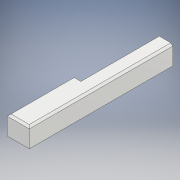
# Autodesk Inventor part: key_2
Saved by Autodesk Inventor 2017 (Build 210142000, 142)
## iProperties
Created: 2018-03-15
Part Number: key_2
Material: Generic
Document SubType Name: Modeling
Designer: Luiz Gustavo
Density: 1 g/cm^3
Appearance: White
Author: Luiz Gustavo
Autodesk Inventor part; units mm, degrees
ref_plane "YZ Plane" through (0, 0, 0) normal (1, 0, 0) x (0, 1, 0)
ref_plane "XZ Plane" through (0, 0, 0) normal (0, 1, 0) x (-1, 0, 0)
ref_plane "XY Plane" through (0, 0, 0) normal (0, 0, 1) x (1, 0, 0)
sketch "Sketch1" plane through (0, 0, 0) normal (0, 0, 1) x (1, 0, 0)
  line L0 (-11.5, -75) -> (11.5, -75)
  line L1 (11.5, -75) -> (11.5, 75)
  line L2 (11.5, 75) -> (-11.5, 75)
  line L3 (-11.5, 75) -> (-11.5, -75)
  line L4 (-11.5, -75) -> (11.5, 75) construction
  line L5 (11.5, -75) -> (-11.5, 75) construction
  line L6 (-11.5, 75) -> (-4.5, 75)
  line L7 (-4.5, 75) -> (-4.5, -5)
  line L8 (-4.5, -5) -> (-11.5, -5)
  line L9 (-11.5, -5) -> (-11.5, 75)
  point P0 (0, 0)
  dimension "d0" = 23
  dimension "d1" = 150
  dimension "d2" = 7
  dimension "d3" = 80
  constraints: 20 end point, 4 parallel, 2 horizontal, 2 midpoint, 2 perpendicular
  measures "d0" distance of L0.start L0.end
  measures "d1" distance between parallel lines of L0 L2
  measures "d2" distance of L7.end L8.end
  measures "d3" distance between parallel lines of L8 L2
extrude "Extrusion1" add sketch "Sketch1" against normal blind 20 contours L3 L8 L7 L2 L1 L0
chamfer "Chamfer1" distance 2 angle 45 5 edges at (0, -75, 0) (-11.5, -40, 0) (11.5, 0, 0) (-8, -5, 0) (-4.5, 35, 0)
equation "\"d0\" = key_width"
equation "\"d1\" = key_length"
equation "\"d2\" = blackkey_halfwidth"
equation "\"d3\" = blackkey_length"
equation "\"d4\" = key_height"
equation "\"key_width\" = 23"
equation "\"key_length\" = 150"
equation "\"blackkey_halfwidth\" = 7"
equation "\"blackkey_length\" = 80"
equation "\"key_height\" = 20"
body "Solid1"
